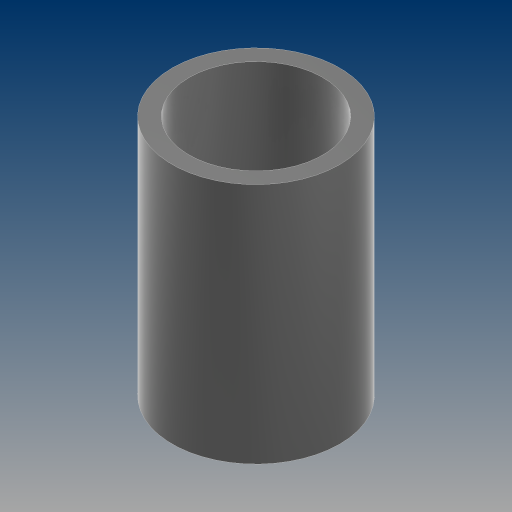
# Autodesk Inventor part: ELEV_040_SPACER12
Saved by Autodesk Inventor 2024.3 (Build 283343000, 343)
## iProperties
Created: 2024-12-04
Part Number: ELEV_040_SPACER12
Material: ABS Plastic
Document SubType Name: Modeling
Designer: Kenji
Density: 1.06 g/cm^3
Appearance: Smooth - Black
Author: Kenji
Autodesk Inventor part; units mm, degrees
ref_plane "YZ Plane" through (0, 0, 0) normal (1, 0, 0) x (0, 1, 0)
ref_plane "XZ Plane" through (0, 0, 0) normal (0, 1, 0) x (-1, 0, 0)
ref_plane "XY Plane" through (0, 0, 0) normal (0, 0, 1) x (1, 0, 0)
sketch "Sketch1" plane through (0, 0, 0) normal (0, 1, 0) x (-1, 0, 0)
  circle A0 centre (0, 0) radius 7.62
  circle A1 centre (0, 0) radius 9.525
  dimension "d0" = 15.24
  dimension "d1" = 19.05
  constraints: 2 centre point, 2 coincident
  measures "d0" diameter of A0
  measures "d1" diameter of A1
extrude "Extrusion1" add sketch "Sketch1" along normal blind 27.5336
body "Solid1"
